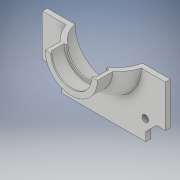
# Autodesk Inventor part: 20_Cube_Insert_Eye_Lens_v3
Saved by Autodesk Inventor 2019 (Build 230136000, 136)
## iProperties
Created: 2020-02-04
Part Number: 20_Cube_Insert_Eye_Lens_v3
Material: Generic
Document SubType Name: Modeling
Designer: marsikovabarbora
Density: 1 g/cm^3
Appearance: Default
Author: marsikovabarbora
Autodesk Inventor part; units mm, degrees
ref_plane "YZ Plane" through (0, 0, 0) normal (1, 0, 0) x (0, 1, 0)
ref_plane "XZ Plane" through (0, 0, 0) normal (0, 1, 0) x (-1, 0, 0)
ref_plane "XY Plane" through (0, 0, 0) normal (0, 0, 1) x (1, 0, 0)
sketch "Sketch1" plane through (0, 0, 0) normal (0, 0, 1) x (1, 0, 0)
  line L0 (-36.8533, 0) -> (46.8153, 0) construction
  line L1 (0, -29.8808) -> (0, 4.9801) construction
  line L2 (0, 0) -> (24.6516, -24.6516) construction
  line L3 (0, 0) -> (34.8626, 0) construction
  line L4 (0, -24.9006) -> (16.8, -24.9006)
  line L5 (16.8, -24.9006) -> (16.8, -21.2406)
  line L6 (16.8, -21.2406) -> (19.0203, -19.0203)
  line L7 (24.9006, 0) -> (24.9006, -16.8)
  line L8 (24.9006, -16.8) -> (21.2406, -16.8)
  line L9 (21.2406, -16.8) -> (19.0203, -19.0203)
  line L10 (0, 0) -> (-24.6516, -24.6516) construction
  line L11 (0, -24.9006) -> (-16.8, -24.9006)
  line L12 (-16.8, -24.9006) -> (-16.8, -21.2406)
  line L13 (-16.8, -21.2406) -> (-19.0203, -19.0203)
  line L14 (-24.9006, 0) -> (-24.9006, -16.8)
  line L15 (-24.9006, -16.8) -> (-21.2406, -16.8)
  line L16 (-21.2406, -16.8) -> (-19.0203, -19.0203)
  arc A0 (-14, 0) -> (14, 0) centre (0, 0) ccw
  line L17 (0, 0) -> (14, 0) construction
  line L18 (0, 0) -> (-14, 0) construction
  line L19 (-14, 0) -> (-24.9006, 0)
  line L20 (14, 0) -> (24.9006, 0)
  dimension "d0" = 45
  dimension "d1" = 16.8
  dimension "d2" = 3.66
  dimension "d4" = 3.14
  dimension "d5" = 14
  dimension "d6" = 180
  constraints: 38 end point, 10 symmetric about line, 4 point on line, 2 horizontal, 2 perpendicular, 2 point on circle, 1 centre point, 1 coincident, 1 equal length
  measures "d0" angle of L2 L3
  measures "d1" distance of L4.start L4.end
  measures "d2" distance of L4.end L5.end
  measures "d4" distance of L5.end L6.end
  measures "d5" radius of A0
  measures "d6" angle of L18 L17
extrude "Extrusion1" add sketch "Sketch1" along normal blind 5
sketch "Sketch3" plane through (-24.9006, 0, 0) normal (0, 1, 0) x (1, 0, 0)
  line L0 (10.9006, 0) -> (0, 0) construction
  line L1 (0, 0) -> (0, -5) construction
  line L2 (10.9006, -5) -> (0, -5) construction
  line L3 (10.9006, 0) -> (10.9006, -5) construction
  line L4 (38.9006, 0) -> (10.9006, 0) construction
  line L5 (10.9006, 0) -> (10.9006, -5) construction
  line L6 (38.9006, -5) -> (10.9006, -5) construction
  line L7 (38.9006, 0) -> (38.9006, -5) construction
  line L8 (49.8013, 0) -> (38.9006, 0) construction
  line L9 (38.9006, 0) -> (38.9006, -5) construction
  line L10 (49.8013, -5) -> (38.9006, -5) construction
  line L11 (49.8013, 0) -> (49.8013, -5) construction
  line L12 (24.9006, 18.5006) -> (24.9006, -23.5037) construction
  arc A0 (10.9006, 0) -> (24.9006, -14) centre (24.9006, 0) ccw
  arc A1 (8.9006, 0) -> (24.9006, -16) centre (24.9006, 0) ccw
  line L13 (24.9006, -16) -> (24.9006, -14)
  line L14 (10.9006, 0) -> (0, 0) projected
  line L15 (8.9006, 0) -> (10.9006, 0)
  dimension "d11" = 2
  constraints: 4 end point, 4 point on circle, 2 centre point, 1 coincident, 1 collinear, 1 horizontal, 1 point on line
  measures "d11" radial gap between concentric circles of A0 A1
revolve "Revolution2" add sketch "Sketch3" angle 180 about axis through (0, 0, -10) along (0, 0, 1)
ref_plane "Work Plane1" through (0, 0, 16) normal (0, 0, 1) x (1, 0, 0)
sketch "Sketch5" plane through (24.9006, 0, 5) normal (0, 1, 0) x (1, 0, 0)
  line L0 (0, 0) -> (-9.7019, 0) construction
  line L1 (0, 5) -> (0, 0) construction
  line L2 (0, 5) -> (-10.9006, 5) construction
  arc A0 (-38.9006, 5) -> (-10.9006, 5) centre (-24.9006, 5) ccw construction
  line L3 (-38.9006, 5) -> (-49.8013, 5) construction
  line L4 (-49.8013, 5) -> (-49.8013, 0) construction
  line L5 (-40.0993, 0) -> (-49.8013, 0) construction
  arc A1 (-40.0993, 0) -> (-9.7019, 0) centre (-24.9006, 5) ccw construction
  arc A2 (-38.9006, 5) -> (-10.9006, 5) centre (-24.9006, 5) ccw construction
  line L6 (-10.9006, 5) -> (-38.9006, 5) construction
  line L7 (-24.9006, 25) -> (-24.9006, -17) construction
  line L8 (-24.9006, -7) -> (-34.0006, -7)
  line L9 (-34.0006, -7) -> (-34.0006, -12.35)
  line L10 (-34.0006, -12.35) -> (-24.9006, -12.35)
  line L11 (-24.9006, -12.35) -> (-24.9006, -7)
  arc A3 (-10.9006, 5) -> (-38.9006, 5) centre (-24.9006, 5) ccw construction
  line L12 (-24.9006, 19) -> (-24.9006, -7) construction
  line L13 (-24.9006, 19) -> (1.0994, 19) construction
  line L14 (-33.0006, -7) -> (-32.1117, -7)
  line L15 (-32.1117, -7) -> (-32.1117, -6.4188)
  line L16 (-32.1117, -6.4188) -> (-33.0006, -6.4188)
  line L17 (-33.0006, -6.4188) -> (-33.0006, -7)
  arc A4 (-38.9006, 5) -> (-10.9006, 5) centre (-24.9006, 5) ccw projected
  line L18 (-24.9006, -12.35) -> (-32.213, -12.35)
  line L19 (-24.9006, -14.25) -> (-24.9006, -12.35)
  arc A5 (-40.0993, 0) -> (-9.7019, 0) centre (-24.9006, 5) ccw projected
  dimension "d16" = 9.1
  dimension "d17" = 5.35
  dimension "d19" = 26
  dimension "d20" = 90
  dimension "d21" = 1
  constraints: 24 end point, 5 point on circle, 4 horizontal, 4 parallel, 3 perpendicular, 3 point on line, 1 centre point, 1 collinear, 1 other
  measures "d16" distance of L8.start L8.end
  measures "d17" distance of L8.end L9.end
  measures "d19" distance of L12.start L12.end
  measures "d20" angle of L12 L13
  measures "d21" distance between parallel lines of L9 L17
revolve "Revolution3" cut sketch "Sketch5" angle 360 about axis through (0, 0, -10) along (0, 0, 1)
sketch "Sketch6" plane through (-24.9006, 0, 5) normal (0, 1, 0) x (1, 0, 0)
  line L0 (15.8006, -8.1602) -> (15.8006, -7) construction
  line L1 (15.8006, -7) -> (16.8006, -7) construction
  line L2 (16.8006, -7) -> (16.8006, -6.4188) construction
  arc A0 (10.9006, 5) -> (16.8006, -6.4188) centre (24.9006, 5) ccw construction
  line L3 (10.9006, 5) -> (0, 5) construction
  line L4 (0, 5) -> (0, 0) construction
  line L5 (9.7019, 0) -> (0, 0) construction
  arc A1 (9.7019, 0) -> (15.8006, -8.1602) centre (24.9006, 5) ccw construction
  line L6 (24.9006, 7.4176) -> (24.9006, -9.5058) construction
  arc A2 (9.7019, 0) -> (15.8006, -8.1602) centre (24.9006, 5) ccw projected
  line L7 (14.3176, -7) -> (14.3176, -13.1753)
  line L8 (15.8006, -7) -> (24.9006, -7) construction
  line L9 (24.9006, -7) -> (24.9006, -12.25) construction
  line L10 (24.9006, -12.25) -> (15.8006, -12.25) construction
  line L11 (15.8006, -12.25) -> (15.8006, -7) construction
  line L12 (34.0006, -7) -> (15.8006, -7) construction
  line L13 (15.8006, -7) -> (24.9006, -7) construction
  line L14 (24.9006, -7) -> (24.9006, -14.85) construction
  line L15 (24.9006, -14.85) -> (15.8006, -14.85) construction
  line L16 (15.8006, -14.85) -> (15.8006, -7) construction
  arc A3 (15.8006, -12.25) -> (24.9006, -14.85) centre (24.9006, 2.375) ccw construction
  line L17 (15.8006, -8.1602) -> (15.8006, -12.25)
  line L18 (14.3176, -13.1753) -> (16.6023, -13.1753)
  line L19 (16.6023, -13.1753) -> (16.6023, -12.7193)
  line L20 (16.6023, -12.7193) -> (15.8006, -12.25)
  line L21 (14.3176, -7) -> (15.8006, -7)
  line L22 (34.0006, -8.1602) -> (15.8006, -8.1602) projected
  line L23 (15.8006, -8.1602) -> (15.8006, -7)
  dimension "d38" = 7.85
  dimension "d41" = 5.25
  constraints: 30 end point, 4 horizontal, 4 parallel, 4 perpendicular, 4 point on circle, 2 point on line, 1 centre point, 1 collinear, 1 tangent, 1 vertical
  measures "d38" distance between parallel lines of L15 L8
  measures "d41" distance of L0.end L10.end
revolve "Revolution4" add sketch "Sketch6" angle 180 about axis through (0, 0, -10) along (0, 0, 1) contours A2 L17 L20 L19 L18 L7
sketch "Skizze8" plane through (0, 0, 5) normal (0, 0, 1) x (1, 0, 0)
  arc A0 (-15.1987, 0) -> (15.1987, 0) centre (0, 0) ccw construction
  line L0 (-15.1987, 0) -> (-24.9006, 0) construction
  line L1 (-24.9006, 0) -> (-24.9006, -16.8) construction
  line L2 (-24.9006, -16.8) -> (-21.2406, -16.8) projected
  line L3 (-21.2406, -16.8) -> (-16.8, -21.2406) projected
  line L4 (-16.8, -21.2406) -> (-16.8, -24.9006) projected
  line L5 (-16.8, -24.9006) -> (16.8, -24.9006) construction
  line L6 (16.8, -24.9006) -> (16.8, -21.2406) projected
  line L7 (16.8, -21.2406) -> (21.2406, -16.8) projected
  line L8 (21.2406, -16.8) -> (24.9006, -16.8) projected
  line L9 (24.9006, -16.8) -> (24.9006, 0) construction
  line L10 (24.9006, 0) -> (15.1987, 0) construction
  line L11 (25.1006, 0.2) -> (25.1006, -17) construction
  line L12 (25.1006, -17) -> (21.3235, -17)
  line L13 (21.3235, -17) -> (17, -21.3235)
  line L14 (17, -21.3235) -> (17, -25.1006)
  line L15 (17, -25.1006) -> (-17, -25.1006) construction
  line L16 (-17, -25.1006) -> (-17, -21.3235)
  line L17 (-17, -21.3235) -> (-21.3235, -17)
  line L18 (-21.3235, -17) -> (-25.1006, -17)
  line L19 (-25.1006, -17) -> (-25.1006, 0.2) construction
  line L20 (-25.1006, 0.2) -> (-14.9974, 0.2) construction
  arc A1 (-14.9974, 0.2) -> (14.9974, 0.2) centre (0, 0) ccw construction
  line L21 (14.9974, 0.2) -> (25.1006, 0.2) construction
  line L22 (-24.9006, -16.8) -> (-24.9006, -17)
  line L23 (-16.8, -24.9006) -> (-17, -24.9006)
  line L24 (16.8, -24.9006) -> (-16.8, -24.9006) projected
  line L25 (16.8, -24.9006) -> (17, -24.9006)
  line L26 (24.9006, 0) -> (24.9006, -16.8) projected
  line L27 (24.9006, -16.8) -> (24.9006, -17)
  point P0 (0, 0)
  dimension "d28" = 0.2
  constraints: 30 end point, 5 point on line, 3 perpendicular, 2 point on circle, 1 centre point, 11 other
  measures "d28" distance between parallel lines of L9 L11
extrude "IM_offset" add sketch "Skizze8" against normal up to surface (5 mm away)
sketch "Sketch9" plane through (0, 0, 5) normal (0, 0, 1) x (1, 0, 0)
  arc A0 (-15.1987, 0) -> (15.1987, 0) centre (0, 0) ccw construction
  line L0 (-15.1987, 0) -> (-24.9006, 0) construction
  line L1 (-24.9006, 0) -> (-24.9006, -17) construction
  line L2 (-17, -24.9006) -> (17, -24.9006) construction
  line L3 (24.9006, -17) -> (24.9006, 0) construction
  line L4 (24.9006, 0) -> (15.1987, 0) construction
  line L5 (-24.9006, -17) -> (-21.3235, -17) projected
  line L6 (-21.3235, -17) -> (-17, -21.3235) projected
  line L7 (-17, -21.3235) -> (-17, -24.9006) projected
  line L8 (17, -24.9006) -> (17, -21.3235) projected
  line L9 (17, -21.3235) -> (21.3235, -17) projected
  line L10 (21.3235, -17) -> (24.9006, -17) projected
  point P0 (0, 0)
  point P1 (-16.9, -16.9)
  point P2 (16.8404, -16.8404)
hole "Hole1" at (-16.9, -16.9, 5) at (16.8404, -16.8404, 5) direction (0, 0, -1) diameter 2.7 end through all
sketch "Sketch10" plane through (0, 0, 0) normal (0, 0, -1) x (-1, 0, 0)
  circle A0 centre (16.9, -16.9) radius 1.35 projected
  circle A1 centre (-16.8404, -16.8404) radius 1.35 projected
  line L0 (-24.9006, 0) -> (-14, 0) projected
  line L1 (-24.9006, 0) -> (-24.9006, -17) projected
  line L2 (-24.9006, -17) -> (-21.3235, -17) projected
  line L3 (-21.3235, -17) -> (-17, -21.3235) projected
  line L4 (-17, -21.3235) -> (-17, -24.9006) projected
  line L5 (-17, -24.9006) -> (17, -24.9006) projected
  line L6 (17, -24.9006) -> (17, -21.3235) projected
  line L7 (17, -21.3235) -> (21.3235, -17) projected
  line L8 (21.3235, -17) -> (24.9006, -17) projected
  line L9 (24.9006, 0) -> (24.9006, -17) projected
  line L10 (14, 0) -> (24.9006, 0) projected
  arc A2 (-14, 0) -> (14, 0) centre (0, 0) ccw projected
  circle A3 centre (0, 0) radius 14
  constraints: 1 centre point, 1 coincident, 1 concentric
extrude "Extrusion5" cut sketch "Sketch10" against normal blind 3
body "Solid1"
